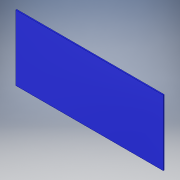
# Autodesk Inventor part: Front
Saved by Autodesk Inventor 2017 (Build 210142000, 142)
## iProperties
Created: 2017-11-22
Part Number: Front
Material: Generic
Document SubType Name: Modeling
Designer: guirguk
Density: 1 g/cm^3
Appearance: Blue - Wall Paint - Glossy
Author: guirguk
Autodesk Inventor part; units mm, degrees
ref_plane "YZ Plane" through (0, 0, 0) normal (1, 0, 0) x (0, 1, 0)
ref_plane "XZ Plane" through (0, 0, 0) normal (0, 1, 0) x (-1, 0, 0)
ref_plane "XY Plane" through (0, 0, 0) normal (0, 0, 1) x (1, 0, 0)
sketch "Sketch1" plane through (0, 0, 0) normal (0, 0, 1) x (1, 0, 0)
  line L0 (0, 0) -> (450.85, 0)
  line L1 (450.85, 0) -> (450.85, 200.025)
  line L2 (450.85, 200.025) -> (0, 200.025)
  line L3 (0, 200.025) -> (0, 0)
  dimension "d1" = 450.85
  dimension "d2" = 200.025
  dimension "d3" = 450.85
  constraints: 8 end point, 2 perpendicular, 1 horizontal
  measures "d1" distance of L0.start L0.end
  measures "d2" distance of L0.end L1.end
  measures "d3" distance of L1.end L2.end
extrude "Extrusion1" add sketch "Sketch1" along normal blind 3.175
body "Solid1"
